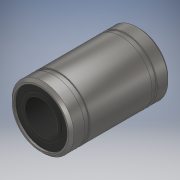
# Autodesk Inventor part: 8mm Linear Bearing
Saved by Autodesk Inventor 2019.1 (Build 231200000, 200)
## iProperties
Created: 2018-08-19
Part Number: 8mm Linear Bearing
Material: Stainless Steel
Document SubType Name: Modeling
Designer: Richard
Density: 8 g/cm^3
Appearance: Semi-Polished
Author: Richard
Autodesk Inventor part; units mm, degrees
ref_plane "YZ Plane" through (0, 0, 0) normal (1, 0, 0) x (0, 1, 0)
ref_plane "XZ Plane" through (0, 0, 0) normal (0, 1, 0) x (-1, 0, 0)
ref_plane "XY Plane" through (0, 0, 0) normal (0, 0, 1) x (1, 0, 0)
sketch "Sketch1" plane through (0, 0, 0) normal (1, 0, 0) x (0, 1, 0)
  line L0 (4, 11.492) -> (4, -11.492)
  line L1 (4, -11.492) -> (6.484, -11.492)
  line L2 (6.484, -11.492) -> (6.484, -12)
  line L3 (6.484, -12) -> (7.5, -12)
  line L4 (7.5, -12) -> (7.5, -8.75)
  line L5 (7.5, -8.75) -> (7.246, -8.75)
  line L6 (7.246, -8.75) -> (7.246, -7.5)
  line L7 (7.246, -7.5) -> (7.5, -7.5)
  line L8 (7.5, -7.5) -> (7.5, 7.5)
  line L9 (7.5, 7.5) -> (7.246, 7.5)
  line L10 (7.246, 7.5) -> (7.246, 8.75)
  line L11 (7.246, 8.75) -> (7.5, 8.75)
  line L12 (7.5, 8.75) -> (7.5, 12)
  line L13 (7.5, 12) -> (6.484, 12)
  line L14 (6.484, 12) -> (6.484, 11.492)
  line L15 (6.484, 11.492) -> (4, 11.492)
  line L16 (0, 0) -> (0, -1.7143)
  line L17 (4, 11.492) -> (4, 11.746)
  line L18 (4, 11.746) -> (4.762, 11.746)
  line L19 (4.762, 11.746) -> (4.762, 11.492)
  line L20 (4, -11.492) -> (4, -11.746)
  line L21 (4, -11.746) -> (4.762, -11.746)
  line L22 (4.762, -11.746) -> (4.762, -11.492)
  point P0 (4, 0)
  point P1 (7.5, 0)
  dimension "d0" = 8
  dimension "d1" = 15
  dimension "d2" = 24
  dimension "d3" = 1.016
  dimension "d4" = 0.254
  dimension "d5" = 0.762
  dimension "d6" = 0.508
  dimension "d7" = 1.25
  dimension "d8" = 0.254
  dimension "d9" = 15
  constraints: 46 end point, 15 perpendicular, 10 point on line, 4 equal length, 4 vertical, 2 horizontal alignment, 2 midpoint
  measures "d0" diameter of L0 L16
  measures "d1" diameter of L8 L16
  measures "d2" distance between parallel lines of L3 L13
  measures "d3" distance of L12.end L13.end
  measures "d4" distance between parallel lines of L18 L13
  measures "d5" distance of L17.end L18.end
  measures "d6" distance of L13.end L14.end
  measures "d7" distance of L9.end L10.end
  measures "d8" distance of L8.end L9.end
  measures "d9" distance of L7.end L8.end
revolve "Revolution1" add sketch "Sketch1" angle 360 about axis through (0, 0, 0) along (0, 0, -1)
chamfer "Chamfer1" distance 0.635 angle 45 2 edges at (0, -7.5, 12) (0, -7.5, -12)
body "Solid1"
